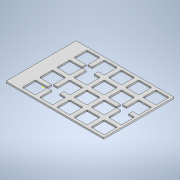
# Autodesk Inventor part: plate
Saved by Autodesk Inventor 2021 (Build 250183000, 183)
## iProperties
Created: 2020-07-21
Part Number: plate
Material: Generic
Document SubType Name: Modeling
Designer: Fireo
Density: 1 g/cm^3
Appearance: Default
Author: Fireo
## iProperties of the stored document _3DPrint.ipt
Created: 2020-07-21
Part Number: _3DPrint
Material: Generic
Document SubType Name: Modeling
Designer: Fireo
Density: 1 g/cm^3
Appearance: Default
Author: Fireo
Autodesk Inventor part; units mm, degrees
ref_plane "YZ Plane" through (0, 0, 0) normal (1, 0, 0) x (0, 1, 0)
ref_plane "XZ Plane" through (0, 0, 0) normal (0, 1, 0) x (-1, 0, 0)
ref_plane "XY Plane" through (0, 0, 0) normal (0, 0, 1) x (1, 0, 0)
sketch "Sketch2" plane through (0, 0, 0) normal (0, 1, 0) x (-1, 0, 0)
  point P0 (0, 0)
sketch "Sketch1" plane through (0, 0, 0) normal (0, 1, 0) x (-1, 0, 0)
  line L0 (8.6807, 13.4166) -> (-3.8693, 13.4166)
  line L1 (-4.8693, 12.4166) -> (-4.8693, -0.1334)
  line L2 (-3.8693, -1.1334) -> (8.6807, -1.1334)
  line L3 (9.6807, -0.1334) -> (9.6807, 12.4166)
  line L4 (8.6807, -20.2334) -> (-3.8693, -20.2334)
  line L5 (-4.8693, -19.2334) -> (-4.8693, -6.6834)
  line L6 (-3.8693, -5.6834) -> (8.6807, -5.6834)
  line L7 (9.6807, -6.6834) -> (9.6807, -19.2334)
  line L8 (8.6807, -58.4334) -> (-3.8693, -58.4334)
  line L9 (-4.8693, -57.4334) -> (-4.8693, -44.8834)
  line L10 (-3.8693, -43.8834) -> (8.6807, -43.8834)
  line L11 (9.6807, -44.8834) -> (9.6807, -57.4334)
  line L12 (8.6807, -24.7834) -> (-3.8693, -24.7834)
  line L13 (-4.8693, -25.7834) -> (-4.8693, -38.3334)
  line L14 (-3.8693, -39.3334) -> (8.6807, -39.3334)
  line L15 (9.6807, -38.3334) -> (9.6807, -25.7834)
  line L16 (-22.9693, 13.4166) -> (-10.4193, 13.4166)
  line L17 (-9.4193, 12.4166) -> (-9.4193, -0.1334)
  line L18 (-10.4193, -1.1334) -> (-22.9693, -1.1334)
  line L19 (-23.9693, -0.1334) -> (-23.9693, 12.4166)
  line L20 (-22.9693, -20.2334) -> (-10.4193, -20.2334)
  line L21 (-9.4193, -19.2334) -> (-9.4193, -6.6834)
  line L22 (-10.4193, -5.6834) -> (-22.9693, -5.6834)
  line L23 (-23.9693, -6.6834) -> (-23.9693, -19.2334)
  line L24 (-22.9693, -58.4334) -> (-10.4193, -58.4334)
  line L25 (-9.4193, -57.4334) -> (-9.4193, -44.8834)
  line L26 (-10.4193, -43.8834) -> (-22.9693, -43.8834)
  line L27 (-23.9693, -44.8834) -> (-23.9693, -57.4334)
  line L28 (-22.9693, -24.7834) -> (-10.4193, -24.7834)
  line L29 (-9.4193, -25.7834) -> (-9.4193, -38.3334)
  line L30 (-10.4193, -39.3334) -> (-22.9693, -39.3334)
  line L31 (-23.9693, -38.3334) -> (-23.9693, -25.7834)
  line L32 (-61.1693, 13.4166) -> (-48.6193, 13.4166)
  line L33 (-47.6193, 12.4166) -> (-47.6193, -0.1334)
  line L34 (-48.6193, -1.1334) -> (-61.1693, -1.1334)
  line L35 (-62.1693, -0.1334) -> (-62.1693, 12.4166)
  line L36 (-61.1693, -20.2334) -> (-48.6193, -20.2334)
  line L37 (-47.6193, -19.2334) -> (-47.6193, -6.6834)
  line L38 (-48.6193, -5.6834) -> (-61.1693, -5.6834)
  line L39 (-62.1693, -6.6834) -> (-62.1693, -19.2334)
  line L40 (-61.1693, -58.4334) -> (-48.6193, -58.4334)
  line L41 (-47.6193, -57.4334) -> (-47.6193, -44.8834)
  line L42 (-48.6193, -43.8834) -> (-61.1693, -43.8834)
  line L43 (-62.1693, -44.8834) -> (-62.1693, -57.4334)
  line L44 (-61.1693, -24.7834) -> (-48.6193, -24.7834)
  line L45 (-47.6193, -25.7834) -> (-47.6193, -38.3334)
  line L46 (-48.6193, -39.3334) -> (-61.1693, -39.3334)
  line L47 (-62.1693, -38.3334) -> (-62.1693, -25.7834)
  line L48 (-29.5193, -24.7834) -> (-42.0693, -24.7834)
  line L49 (-43.0693, -25.7834) -> (-43.0693, -38.3334)
  line L50 (-42.0693, -39.3334) -> (-29.5193, -39.3334)
  line L51 (-28.5193, -38.3334) -> (-28.5193, -25.7834)
  line L52 (-42.0693, -43.8834) -> (-29.5193, -43.8834)
  line L53 (-29.5193, -58.4334) -> (-42.0693, -58.4334)
  line L54 (-28.5193, -44.8834) -> (-28.5193, -57.4334)
  line L55 (-43.0693, -57.4334) -> (-43.0693, -44.8834)
  line L56 (-29.5193, 13.4166) -> (-42.0693, 13.4166)
  line L57 (-43.0693, -19.2334) -> (-43.0693, -6.6834)
  line L58 (-42.0693, -5.6834) -> (-29.5193, -5.6834)
  line L59 (-28.5193, -6.6834) -> (-28.5193, -19.2334)
  line L60 (-42.0693, -1.1334) -> (-29.5193, -1.1334)
  line L61 (-43.0693, 12.4166) -> (-43.0693, -0.1334)
  line L62 (-28.5193, -0.1334) -> (-28.5193, 12.4166)
  line L63 (-29.5193, -20.2334) -> (-42.0693, -20.2334)
  line L64 (-81.2693, -25.7834) -> (-81.2693, -38.3334)
  line L65 (-80.2693, -1.1334) -> (-67.7193, -1.1334)
  line L66 (-81.2693, 12.4166) -> (-81.2693, -0.1334)
  line L67 (-67.7193, 13.4166) -> (-80.2693, 13.4166)
  line L68 (-66.7193, -0.1334) -> (-66.7193, 12.4166)
  line L69 (-67.7193, -20.2334) -> (-80.2693, -20.2334)
  line L70 (-81.2693, -19.2334) -> (-81.2693, -6.6834)
  line L71 (-80.2693, -5.6834) -> (-67.7193, -5.6834)
  line L72 (-66.7193, -6.6834) -> (-66.7193, -19.2334)
  line L73 (-67.7193, -24.7834) -> (-80.2693, -24.7834)
  line L74 (-66.7193, -38.3334) -> (-66.7193, -25.7834)
  line L75 (-80.2693, -39.3334) -> (-67.7193, -39.3334)
  line L76 (-81.2693, -57.4334) -> (-81.2693, -44.8834)
  line L77 (-67.7193, -58.4334) -> (-80.2693, -58.4334)
  line L78 (-66.7193, -44.8834) -> (-66.7193, -57.4334)
  line L79 (-80.2693, -43.8834) -> (-67.7193, -43.8834)
  arc A0 (9.6807, 12.4166) -> (8.6807, 13.4166) centre (8.6807, 12.4166) ccw
  arc A1 (-3.8693, 13.4166) -> (-4.8693, 12.4166) centre (-3.8693, 12.4166) ccw
  arc A2 (8.6807, -1.1334) -> (9.6807, -0.1334) centre (8.6807, -0.1334) ccw
  arc A3 (-4.8693, -0.1334) -> (-3.8693, -1.1334) centre (-3.8693, -0.1334) ccw
  arc A4 (-9.4193, 12.4166) -> (-10.4193, 13.4166) centre (-10.4193, 12.4166) ccw
  arc A5 (-23.9693, -0.1334) -> (-22.9693, -1.1334) centre (-22.9693, -0.1334) ccw
  arc A6 (-22.9693, 13.4166) -> (-23.9693, 12.4166) centre (-22.9693, 12.4166) ccw
  arc A7 (-10.4193, -1.1334) -> (-9.4193, -0.1334) centre (-10.4193, -0.1334) ccw
  arc A8 (9.6807, -6.6834) -> (8.6807, -5.6834) centre (8.6807, -6.6834) ccw
  arc A9 (-3.8693, -5.6834) -> (-4.8693, -6.6834) centre (-3.8693, -6.6834) ccw
  arc A10 (-4.8693, -19.2334) -> (-3.8693, -20.2334) centre (-3.8693, -19.2334) ccw
  arc A11 (8.6807, -20.2334) -> (9.6807, -19.2334) centre (8.6807, -19.2334) ccw
  arc A12 (9.6807, -25.7834) -> (8.6807, -24.7834) centre (8.6807, -25.7834) ccw
  arc A13 (-4.8693, -38.3334) -> (-3.8693, -39.3334) centre (-3.8693, -38.3334) ccw
  arc A14 (8.6807, -39.3334) -> (9.6807, -38.3334) centre (8.6807, -38.3334) ccw
  arc A15 (-3.8693, -24.7834) -> (-4.8693, -25.7834) centre (-3.8693, -25.7834) ccw
  arc A16 (-3.8693, -43.8834) -> (-4.8693, -44.8834) centre (-3.8693, -44.8834) ccw
  arc A17 (9.6807, -44.8834) -> (8.6807, -43.8834) centre (8.6807, -44.8834) ccw
  arc A18 (8.6807, -58.4334) -> (9.6807, -57.4334) centre (8.6807, -57.4334) ccw
  arc A19 (-4.8693, -57.4334) -> (-3.8693, -58.4334) centre (-3.8693, -57.4334) ccw
  arc A20 (-23.9693, -19.2334) -> (-22.9693, -20.2334) centre (-22.9693, -19.2334) ccw
  arc A21 (-22.9693, -5.6834) -> (-23.9693, -6.6834) centre (-22.9693, -6.6834) ccw
  arc A22 (-9.4193, -6.6834) -> (-10.4193, -5.6834) centre (-10.4193, -6.6834) ccw
  arc A23 (-10.4193, -20.2334) -> (-9.4193, -19.2334) centre (-10.4193, -19.2334) ccw
  arc A24 (-22.9693, -24.7834) -> (-23.9693, -25.7834) centre (-22.9693, -25.7834) ccw
  arc A25 (-9.4193, -25.7834) -> (-10.4193, -24.7834) centre (-10.4193, -25.7834) ccw
  arc A26 (-10.4193, -39.3334) -> (-9.4193, -38.3334) centre (-10.4193, -38.3334) ccw
  arc A27 (-23.9693, -38.3334) -> (-22.9693, -39.3334) centre (-22.9693, -38.3334) ccw
  arc A28 (-22.9693, -43.8834) -> (-23.9693, -44.8834) centre (-22.9693, -44.8834) ccw
  arc A29 (-9.4193, -44.8834) -> (-10.4193, -43.8834) centre (-10.4193, -44.8834) ccw
  arc A30 (-10.4193, -58.4334) -> (-9.4193, -57.4334) centre (-10.4193, -57.4334) ccw
  arc A31 (-23.9693, -57.4334) -> (-22.9693, -58.4334) centre (-22.9693, -57.4334) ccw
  arc A32 (-43.0693, -19.2334) -> (-42.0693, -20.2334) centre (-42.0693, -19.2334) ccw
  arc A33 (-42.0693, -24.7834) -> (-43.0693, -25.7834) centre (-42.0693, -25.7834) ccw
  arc A34 (-29.5193, -20.2334) -> (-28.5193, -19.2334) centre (-29.5193, -19.2334) ccw
  arc A35 (-28.5193, -25.7834) -> (-29.5193, -24.7834) centre (-29.5193, -25.7834) ccw
  arc A36 (-29.5193, -1.1334) -> (-28.5193, -0.1334) centre (-29.5193, -0.1334) ccw
  arc A37 (-28.5193, -6.6834) -> (-29.5193, -5.6834) centre (-29.5193, -6.6834) ccw
  arc A38 (-28.5193, 12.4166) -> (-29.5193, 13.4166) centre (-29.5193, 12.4166) ccw
  arc A39 (-42.0693, 13.4166) -> (-43.0693, 12.4166) centre (-42.0693, 12.4166) ccw
  arc A40 (-47.6193, 12.4166) -> (-48.6193, 13.4166) centre (-48.6193, 12.4166) ccw
  arc A41 (-61.1693, 13.4166) -> (-62.1693, 12.4166) centre (-61.1693, 12.4166) ccw
  arc A42 (-66.7193, 12.4166) -> (-67.7193, 13.4166) centre (-67.7193, 12.4166) ccw
  arc A43 (-80.2693, 13.4166) -> (-81.2693, 12.4166) centre (-80.2693, 12.4166) ccw
  arc A44 (-81.2693, -57.4334) -> (-80.2693, -58.4334) centre (-80.2693, -57.4334) ccw
  arc A45 (-67.7193, -58.4334) -> (-66.7193, -57.4334) centre (-67.7193, -57.4334) ccw
  arc A46 (-62.1693, -57.4334) -> (-61.1693, -58.4334) centre (-61.1693, -57.4334) ccw
  arc A47 (-48.6193, -58.4334) -> (-47.6193, -57.4334) centre (-48.6193, -57.4334) ccw
  arc A48 (-43.0693, -57.4334) -> (-42.0693, -58.4334) centre (-42.0693, -57.4334) ccw
  arc A49 (-29.5193, -58.4334) -> (-28.5193, -57.4334) centre (-29.5193, -57.4334) ccw
  arc A50 (-29.5193, -39.3334) -> (-28.5193, -38.3334) centre (-29.5193, -38.3334) ccw
  arc A51 (-28.5193, -44.8834) -> (-29.5193, -43.8834) centre (-29.5193, -44.8834) ccw
  arc A52 (-43.0693, -38.3334) -> (-42.0693, -39.3334) centre (-42.0693, -38.3334) ccw
  arc A53 (-42.0693, -43.8834) -> (-43.0693, -44.8834) centre (-42.0693, -44.8834) ccw
  arc A54 (-61.1693, -43.8834) -> (-62.1693, -44.8834) centre (-61.1693, -44.8834) ccw
  arc A55 (-62.1693, -38.3334) -> (-61.1693, -39.3334) centre (-61.1693, -38.3334) ccw
  arc A56 (-48.6193, -39.3334) -> (-47.6193, -38.3334) centre (-48.6193, -38.3334) ccw
  arc A57 (-47.6193, -44.8834) -> (-48.6193, -43.8834) centre (-48.6193, -44.8834) ccw
  arc A58 (-66.7193, -44.8834) -> (-67.7193, -43.8834) centre (-67.7193, -44.8834) ccw
  arc A59 (-80.2693, -43.8834) -> (-81.2693, -44.8834) centre (-80.2693, -44.8834) ccw
  arc A60 (-81.2693, -38.3334) -> (-80.2693, -39.3334) centre (-80.2693, -38.3334) ccw
  arc A61 (-67.7193, -39.3334) -> (-66.7193, -38.3334) centre (-67.7193, -38.3334) ccw
  arc A62 (-66.7193, -25.7834) -> (-67.7193, -24.7834) centre (-67.7193, -25.7834) ccw
  arc A63 (-42.0693, -5.6834) -> (-43.0693, -6.6834) centre (-42.0693, -6.6834) ccw
  arc A64 (-43.0693, -0.1334) -> (-42.0693, -1.1334) centre (-42.0693, -0.1334) ccw
  arc A65 (-62.1693, -0.1334) -> (-61.1693, -1.1334) centre (-61.1693, -0.1334) ccw
  arc A66 (-48.6193, -1.1334) -> (-47.6193, -0.1334) centre (-48.6193, -0.1334) ccw
  arc A67 (-47.6193, -6.6834) -> (-48.6193, -5.6834) centre (-48.6193, -6.6834) ccw
  arc A68 (-61.1693, -5.6834) -> (-62.1693, -6.6834) centre (-61.1693, -6.6834) ccw
  arc A69 (-62.1693, -19.2334) -> (-61.1693, -20.2334) centre (-61.1693, -19.2334) ccw
  arc A70 (-48.6193, -20.2334) -> (-47.6193, -19.2334) centre (-48.6193, -19.2334) ccw
  arc A71 (-47.6193, -25.7834) -> (-48.6193, -24.7834) centre (-48.6193, -25.7834) ccw
  arc A72 (-61.1693, -24.7834) -> (-62.1693, -25.7834) centre (-61.1693, -25.7834) ccw
  arc A73 (-67.7193, -20.2334) -> (-66.7193, -19.2334) centre (-67.7193, -19.2334) ccw
  arc A74 (-81.2693, -19.2334) -> (-80.2693, -20.2334) centre (-80.2693, -19.2334) ccw
  arc A75 (-80.2693, -5.6834) -> (-81.2693, -6.6834) centre (-80.2693, -6.6834) ccw
  arc A76 (-81.2693, -0.1334) -> (-80.2693, -1.1334) centre (-80.2693, -0.1334) ccw
  arc A77 (-67.7193, -1.1334) -> (-66.7193, -0.1334) centre (-67.7193, -0.1334) ccw
  arc A78 (-66.7193, -6.6834) -> (-67.7193, -5.6834) centre (-67.7193, -6.6834) ccw
  arc A79 (-80.2693, -24.7834) -> (-81.2693, -25.7834) centre (-80.2693, -25.7834) ccw
  line L80 (24.6807, 16.4166) -> (24.6807, -61.4334)
  line L81 (24.6807, 16.4166) -> (-83.7693, 16.4166)
  line L82 (24.6807, -61.4334) -> (-83.7693, -61.4334)
  line L83 (-83.7693, 16.4166) -> (-83.7693, -61.4334)
  line L84 (-3.8693, -38.3334) -> (-17.3943, -38.3334)
  line L85 (-17.3943, -38.3334) -> (-17.3943, -44.8834)
  line L86 (-17.3943, -44.8834) -> (-3.8693, -44.8834)
  line L87 (-3.8693, -44.8834) -> (-3.8693, -38.3334)
  line L88 (-3.8693, -0.1334) -> (-17.3943, -0.1334)
  line L89 (-17.3943, -0.1334) -> (-17.3943, -6.6834)
  line L90 (-17.3943, -6.6834) -> (-3.8693, -6.6834)
  line L91 (-3.8693, -6.6834) -> (-3.8693, -0.1334)
  line L92 (-61.1693, -19.2334) -> (-74.6943, -19.2334)
  line L93 (-74.6943, -19.2334) -> (-74.6943, -25.7834)
  line L94 (-74.6943, -25.7834) -> (-61.1693, -25.7834)
  line L95 (-61.1693, -25.7834) -> (-61.1693, -19.2334)
  point P0 (0, 0)
  point P1 (-4.8693, -1.1334)
  point P2 (-4.8693, 13.4166)
  point P3 (9.6807, -1.1334)
  point P4 (0, -5.6169)
  point P5 (0, -45.0169)
  point P6 (0, -39.4)
  point P7 (-10.2886, 0)
  point P8 (-10.2886, -5.6169)
  point P9 (-10.2886, -45.0169)
  point P10 (-10.2886, -39.4)
  point P11 (-49.6886, 0)
  point P12 (-49.6886, -5.6169)
  point P13 (-49.6886, -45.0169)
  point P14 (-49.6886, -39.4)
  point P15 (-39.4, -39.4)
  point P16 (-39.4, -45.0169)
  point P17 (-39.4, 0)
  point P18 (-39.4, -5.6169)
  point P19 (-78.8, 0)
  point P20 (-78.8, -5.6169)
  point P21 (-78.8, -45.0169)
  point P22 (-78.8, -39.4)
  point P23 (-66.7193, -25.7834)
  point P24 (-74.6943, -24.7834)
  point P25 (-74.6943, -20.2334)
  point P26 (-66.7193, -19.2334)
  point P27 (-62.1693, -19.2334)
  point P28 (-61.1693, -24.7834)
  point P29 (-17.3943, -43.8834)
  point P30 (-17.3943, -39.3334)
  point P31 (-3.8693, -43.8834)
  point P32 (-3.8693, -1.1334)
  point P33 (-3.8693, -5.6834)
  point P34 (-4.8693, -6.6834)
  point P35 (-9.4193, -6.6834)
  point P36 (-17.3943, -5.6834)
  point P37 (-17.3943, -1.1334)
  point P38 (-9.4193, -0.1334)
  point P39 (-4.8693, -0.1334)
  point P40 (-3.8693, -39.3334)
  point P41 (-4.8693, -38.3334)
  point P42 (-3.8693, -43.8834)
  point P43 (-66.7193, -25.7834)
  point P44 (-61.1693, -20.2334)
  point P45 (-62.1693, -19.2334)
  point P46 (-61.1693, -24.7834)
  point P47 (-3.8693, -5.6834)
  point P48 (-9.4193, -6.6834)
  point P49 (-4.8693, -6.6834)
  point P50 (-3.8693, -1.1334)
  point P51 (-4.8693, -0.1334)
  point P52 (-9.4193, -0.1334)
  dimension "d0" = 14.55
  dimension "d1" = 14.55
  dimension "d7" = 1
  dimension "d8" = 1
  dimension "d9" = 1
  dimension "d10" = 15
  dimension "d11" = 3
  dimension "d13" = 2.5
  dimension "d17" = 14.55
  dimension "d18" = 14.55
  dimension "d19" = 14.55
  dimension "d20" = 4.55
  dimension "d21" = 4.55
  dimension "d22" = 14.55
  dimension "d23" = 14.55
  dimension "d24" = 4.55
  dimension "d25" = 4.55
  dimension "d26" = 4.55
  dimension "d27" = 4.55
  dimension "d28" = 4.55
  dimension "d29" = 4.55
  dimension "d30" = 4.55
  dimension "d31" = 4.55
  dimension "d32" = 4.55
  dimension "d33" = 4.55
  dimension "d34" = 4.55
  dimension "d35" = 4.55
  dimension "d36" = 4.55
  dimension "d37" = 4.55
  dimension "d38" = 4.55
  dimension "d39" = 4.55
  dimension "d40" = 4.55
  dimension "d41" = 4.55
  dimension "d42" = 4.55
  dimension "d43" = 4.55
  dimension "d44" = 4.55
  dimension "d45" = 3
  dimension "d46" = 3
  dimension "d48" = 3
  dimension "d49" = 3
  dimension "d50" = 3
  dimension "d51" = 3
  dimension "d52" = 3
  dimension "d53" = 14.55
  dimension "d54" = 14.55
  dimension "d55" = 14.55
  dimension "d56" = 14.55
  dimension "d57" = 14.55
  dimension "d58" = 14.55
  dimension "d59" = 14.55
  dimension "d60" = 14.55
  dimension "d61" = 14.55
  dimension "d62" = 14.55
  dimension "d63" = 14.55
  dimension "d64" = 14.55
  dimension "d65" = 14.55
  dimension "d66" = 14.55
  dimension "d67" = 14.55
  dimension "d69" = 14.55
  dimension "d70" = 14.55
  dimension "d71" = 14.55
  dimension "d72" = 14.55
  dimension "d73" = 14.55
  dimension "d74" = 14.55
  constraints: 192 end point, 160 point on circle, 160 tangent, 80 centre point, 77 equal radius, 8 parallel, 7 point on line, 6 horizontal, 4 perpendicular, 2 vertical
  measures "d0" distance of point (9.681, -1.133) point (-4.869, -1.133)
  measures "d1" distance of point (-4.869, -1.133) point (-4.869, 13.417)
  measures "d7" radius of A0
  measures "d8" radius of A53
  measures "d9" radius of A63
  measures "d10" distance between parallel lines of L7 L80
  measures "d11" distance between parallel lines of L0 L81
  measures "d13" distance between parallel lines of L76 L83
  measures "d17" distance between parallel lines of L4 L6
  measures "d18" distance between parallel lines of L7 L5
  measures "d19" distance between parallel lines of L14 L12
  measures "d20" distance between parallel lines of L12 L4
  measures "d21" distance between parallel lines of L6 L2
  measures "d22" distance between parallel lines of L16 L18
  measures "d23" distance between parallel lines of L19 L17
  measures "d24" distance between parallel lines of L18 L22
  measures "d25" distance between parallel lines of L28 L20
  measures "d26" distance between parallel lines of L26 L30
  measures "d27" distance between parallel lines of L52 L50
  measures "d28" distance between parallel lines of L48 L63
  measures "d29" distance between parallel lines of L58 L60
  measures "d30" distance between parallel lines of L38 L34
  measures "d31" distance between parallel lines of L44 L36
  measures "d32" distance between parallel lines of L42 L46
  measures "d33" distance between parallel lines of L79 L75
  measures "d34" distance between parallel lines of L73 L69
  measures "d35" distance between parallel lines of L71 L65
  measures "d36" distance between parallel lines of L68 L35
  measures "d37" distance between parallel lines of L72 L39
  measures "d38" distance between parallel lines of L78 L43
  measures "d39" distance between parallel lines of L74 L47
  measures "d40" distance between parallel lines of L57 L37
  measures "d41" distance between parallel lines of L33 L61
  measures "d42" distance between parallel lines of L45 L49
  measures "d43" distance between parallel lines of L41 L55
  measures "d44" distance between parallel lines of L54 L27
  measures "d45" distance between parallel lines of L81 L16
  measures "d46" distance between parallel lines of L82 L24
  measures "d48" distance between parallel lines of L82 L40
  measures "d49" distance between parallel lines of L82 L77
  measures "d50" distance between parallel lines of L81 L67
  measures "d51" distance between parallel lines of L81 L32
  measures "d52" distance between parallel lines of L81 L56
  measures "d53" distance between parallel lines of L13 L15
  measures "d54" distance between parallel lines of L9 L11
  measures "d55" distance between parallel lines of L8 L10
  measures "d56" distance between parallel lines of L20 L22
  measures "d57" distance between parallel lines of L21 L23
  measures "d58" distance between parallel lines of L30 L28
  measures "d59" distance between parallel lines of L29 L31
  measures "d60" distance between parallel lines of L24 L26
  measures "d61" distance between parallel lines of L25 L27
  measures "d62" distance between parallel lines of L60 L56
  measures "d63" distance between parallel lines of L61 L62
  measures "d64" distance between parallel lines of L59 L57
  measures "d65" distance between parallel lines of L58 L63
  measures "d66" distance between parallel lines of L50 L48
  measures "d67" distance between parallel lines of L51 L49
  measures "d69" distance between parallel lines of L55 L54
  measures "d70" distance between parallel lines of L46 L44
  measures "d71" distance between parallel lines of L45 L47
  measures "d72" distance between parallel lines of L36 L38
  measures "d73" distance between parallel lines of L37 L39
  measures "d74" distance between parallel lines of L34 L32
extrude "Extrusion2" add sketch "Sketch1" along normal blind 1.6
body "Solid2"
